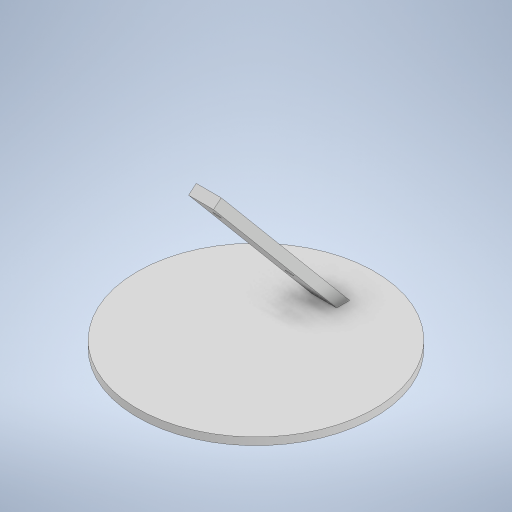
# Autodesk Inventor part: CB_middle_v1
Saved by Autodesk Inventor 2024 (Build 280153000, 153)
## iProperties
Created: 2023-12-13
Part Number: CB_middle_v1
Material: 一般
Document SubType Name: Modeling
Designer: renee
Density: 1 g/cm^3
Appearance: 預設
Author: renee
Autodesk Inventor part; units mm, degrees
ref_plane "YZ Plane" through (0, 0, 0) normal (1, 0, 0) x (0, 1, 0)
ref_plane "XZ Plane" through (0, 0, 0) normal (0, 1, 0) x (-1, 0, 0)
ref_plane "XY Plane" through (0, 0, 0) normal (0, 0, 1) x (1, 0, 0)
sketch "草圖1" plane through (0, 0, 0) normal (0, 1, 0) x (-1, 0, 0)
  circle A0 centre (0, 0) radius 47.5
  dimension "d0" = 95
  constraints: 1 centre point, 1 coincident
  measures "d0" diameter of A0
extrude "擠出1" add sketch "草圖1" along normal blind 3
sketch "草圖2" plane through (0, 0, 0) normal (1, 0, 0) x (0, 1, 0)
  line L0 (3, -47.5) -> (3, 47.5) projected
  line L1 (0, -47.5) -> (0, 47.5) projected
  line L2 (64.2836, 18.923) -> (61.7124, 21.9872)
  line L3 (61.7124, 21.9872) -> (0.4288, -29.4358)
  line L4 (0.4288, -29.4358) -> (3, -32.5)
  line L5 (3, -32.5) -> (64.2836, 18.923)
  point P0 (0, 0)
  dimension "d3" = 4
  dimension "d4" = 80
  dimension "d5" = 50
  dimension "d6" = 15
  constraints: 8 end point, 2 parallel, 1 perpendicular, 1 point on line
  measures "d3" distance between parallel lines of L3 L5
  measures "d4" distance between parallel lines of L4 L2
  measures "d5" angle of L0 L5
  measures "d6" distance of L0.start L4.end
extrude "擠出2" add sketch "草圖2" along normal mid plane 10
sketch "草圖3" plane through (5, 64.2836, 18.923) normal (0, 0.6428, -0.766) x (-1, 0, 0)
  line L0 (10, 0) -> (0, 0) projected
  line L1 (0, -80) -> (0, 0) projected
  line L2 (10, -80) -> (0, -80) projected
  line L3 (10, 0) -> (10, -80) projected
  circle A0 centre (5, -10) radius 1.5
  circle A1 centre (5, -55) radius 1.5
  point P0 (5, -61.4075)
  dimension "d9" = 3
  dimension "d10" = 3
  dimension "d11" = 45
  dimension "d15" = 10
  constraints: 2 centre point, 2 vertical alignment
  measures "d9" diameter of A0
  measures "d10" diameter of A1
  measures "d11" distance of A1.centre A0.centre
  measures "d15" distance from line of A0.centre L0
extrude "擠出3" cut sketch "草圖3" against normal blind 10 contours A0 | A1
